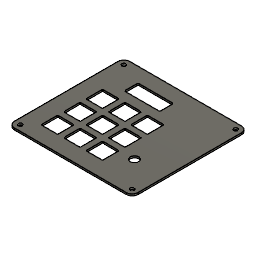
MyMacroPad (Autodesk Fusion 360 archive; units mm, degrees)
design "Top MacroPad"
Autodesk Fusion 360 part; units mm, degrees
sketch "plate-2026-01-30T15_29_04.840Z" plane through (0, 0, 0) normal (0, 0, 1) x (1, 0, 0)
  line L0 (3.025, -21.575) -> (16.025, -21.575)
  line L1 (3.025, -35.575) -> (16.025, -35.575)
  line L2 (2.525, -22.075) -> (2.525, -35.075)
  line L3 (16.525, -22.075) -> (16.525, -35.075)
  arc A0 (3.025, -21.575) -> (2.525, -22.075) centre (3.025, -22.075) ccw
  arc A1 (16.525, -22.075) -> (16.025, -21.575) centre (16.025, -22.075) ccw
  arc A2 (2.525, -35.075) -> (3.025, -35.575) centre (3.025, -35.075) ccw
  arc A3 (16.025, -35.575) -> (16.525, -35.075) centre (16.025, -35.075) ccw
  line L4 (22.075, -21.575) -> (35.075, -21.575)
  line L5 (22.075, -35.575) -> (35.075, -35.575)
  line L6 (21.575, -22.075) -> (21.575, -35.075)
  line L7 (35.575, -22.075) -> (35.575, -35.075)
  arc A4 (22.075, -21.575) -> (21.575, -22.075) centre (22.075, -22.075) ccw
  arc A5 (35.575, -22.075) -> (35.075, -21.575) centre (35.075, -22.075) ccw
  arc A6 (21.575, -35.075) -> (22.075, -35.575) centre (22.075, -35.075) ccw
  arc A7 (35.075, -35.575) -> (35.575, -35.075) centre (35.075, -35.075) ccw
  line L8 (41.125, -21.575) -> (54.125, -21.575)
  line L9 (41.125, -35.575) -> (54.125, -35.575)
  line L10 (40.625, -22.075) -> (40.625, -35.075)
  line L11 (54.625, -22.075) -> (54.625, -35.075)
  arc A8 (41.125, -21.575) -> (40.625, -22.075) centre (41.125, -22.075) ccw
  arc A9 (54.625, -22.075) -> (54.125, -21.575) centre (54.125, -22.075) ccw
  arc A10 (40.625, -35.075) -> (41.125, -35.575) centre (41.125, -35.075) ccw
  arc A11 (54.125, -35.575) -> (54.625, -35.075) centre (54.125, -35.075) ccw
  line L12 (3.025, -40.625) -> (16.025, -40.625)
  line L13 (3.025, -54.625) -> (16.025, -54.625)
  line L14 (2.525, -41.125) -> (2.525, -54.125)
  line L15 (16.525, -41.125) -> (16.525, -54.125)
  arc A12 (3.025, -40.625) -> (2.525, -41.125) centre (3.025, -41.125) ccw
  arc A13 (16.525, -41.125) -> (16.025, -40.625) centre (16.025, -41.125) ccw
  arc A14 (2.525, -54.125) -> (3.025, -54.625) centre (3.025, -54.125) ccw
  arc A15 (16.025, -54.625) -> (16.525, -54.125) centre (16.025, -54.125) ccw
  line L16 (22.075, -40.625) -> (35.075, -40.625)
  line L17 (22.075, -54.625) -> (35.075, -54.625)
  line L18 (21.575, -41.125) -> (21.575, -54.125)
  line L19 (35.575, -41.125) -> (35.575, -54.125)
  arc A16 (22.075, -40.625) -> (21.575, -41.125) centre (22.075, -41.125) ccw
  arc A17 (35.575, -41.125) -> (35.075, -40.625) centre (35.075, -41.125) ccw
  arc A18 (21.575, -54.125) -> (22.075, -54.625) centre (22.075, -54.125) ccw
  arc A19 (35.075, -54.625) -> (35.575, -54.125) centre (35.075, -54.125) ccw
  line L20 (41.125, -40.625) -> (54.125, -40.625)
  line L21 (41.125, -54.625) -> (54.125, -54.625)
  line L22 (40.625, -41.125) -> (40.625, -54.125)
  line L23 (54.625, -41.125) -> (54.625, -54.125)
  arc A20 (41.125, -40.625) -> (40.625, -41.125) centre (41.125, -41.125) ccw
  arc A21 (54.625, -41.125) -> (54.125, -40.625) centre (54.125, -41.125) ccw
  arc A22 (40.625, -54.125) -> (41.125, -54.625) centre (41.125, -54.125) ccw
  arc A23 (54.125, -54.625) -> (54.625, -54.125) centre (54.125, -54.125) ccw
  line L24 (3.025, -59.675) -> (16.025, -59.675)
  line L25 (3.025, -73.675) -> (16.025, -73.675)
  line L26 (2.525, -60.175) -> (2.525, -73.175)
  line L27 (16.525, -60.175) -> (16.525, -73.175)
  arc A24 (3.025, -59.675) -> (2.525, -60.175) centre (3.025, -60.175) ccw
  arc A25 (16.525, -60.175) -> (16.025, -59.675) centre (16.025, -60.175) ccw
  arc A26 (2.525, -73.175) -> (3.025, -73.675) centre (3.025, -73.175) ccw
  arc A27 (16.025, -73.675) -> (16.525, -73.175) centre (16.025, -73.175) ccw
  line L28 (22.075, -59.675) -> (35.075, -59.675)
  line L29 (22.075, -73.675) -> (35.075, -73.675)
  line L30 (21.575, -60.175) -> (21.575, -73.175)
  line L31 (35.575, -60.175) -> (35.575, -73.175)
  arc A28 (22.075, -59.675) -> (21.575, -60.175) centre (22.075, -60.175) ccw
  arc A29 (35.575, -60.175) -> (35.075, -59.675) centre (35.075, -60.175) ccw
  arc A30 (21.575, -73.175) -> (22.075, -73.675) centre (22.075, -73.175) ccw
  arc A31 (35.075, -73.675) -> (35.575, -73.175) centre (35.075, -73.175) ccw
  line L32 (41.125, -59.675) -> (54.125, -59.675)
  line L33 (41.125, -73.675) -> (54.125, -73.675)
  line L34 (40.625, -60.175) -> (40.625, -73.175)
  line L35 (54.625, -60.175) -> (54.625, -73.175)
  arc A32 (41.125, -59.675) -> (40.625, -60.175) centre (41.125, -60.175) ccw
  arc A33 (54.625, -60.175) -> (54.125, -59.675) centre (54.125, -60.175) ccw
  arc A34 (40.625, -73.175) -> (41.125, -73.675) centre (41.125, -73.175) ccw
  arc A35 (54.125, -73.675) -> (54.625, -73.175) centre (54.125, -73.175) ccw
  line L36 (-11.475, 10.56) -> (93.525, 10.56)
  line L37 (93.525, 10.56) -> (93.525, -87.44)
  line L38 (93.525, -87.44) -> (-11.475, -87.44)
  line L39 (-11.475, -87.44) -> (-11.475, 10.56)
  line L40 (13.025, -1.94) -> (43.025, -1.94)
  line L41 (43.025, -1.94) -> (43.025, -13.44)
  line L42 (43.025, -13.44) -> (13.025, -13.44)
  line L43 (13.025, -13.44) -> (13.025, -1.94)
  circle A36 centre (67.525, -59.44) radius 3.55
  circle A37 centre (-6.475, -82.44) radius 1.7
  circle A38 centre (-6.475, 5.56) radius 1.7
  circle A39 centre (88.525, 5.56) radius 1.7
  circle A40 centre (88.525, -82.44) radius 1.7
  dimension "d1" = 98
  dimension "d2" = 105
  dimension "d4" = 14
  dimension "d5" = 13.765
  dimension "d9" = 12.5
  dimension "d13" = 7.1
  dimension "d16" = 3.4
  dimension "d17" = 5
  dimension "d18" = 5
  dimension "d19" = 3.4
  dimension "d20" = 5
  dimension "d21" = 5
  dimension "d22" = 3.4
  dimension "d23" = 5
  dimension "d24" = 5
  dimension "d25" = 3.4
  dimension "d26" = 5
  dimension "d27" = 5
  dimension "d28" = 30
  dimension "d29" = 11.5
  dimension "d56" = 24.5
  dimension "d63" = 28
  dimension "d64" = 26
  constraint horizontal L36
  constraint vertical L37
  constraint horizontal L38
  constraint vertical L39
  constraint horizontal L40
  constraint vertical L41
  constraint horizontal L42
  constraint vertical L43
  measures "d1" distance of L36.start L38.end
  measures "d2" distance of L36.start L36.end
  measures "d4" distance of L26.start L39
  measures "d5" distance of L25.start L38
  measures "d9" distance of L36 L40.start
  measures "d13" diameter of A36
  measures "d16" diameter of A37
  measures "d17" distance of L38 A37.centre
  measures "d18" distance of L39 A37.centre
  measures "d19" diameter of A38
  measures "d20" distance of L36 A38.centre
  measures "d21" distance of L39 A38.centre
  measures "d22" diameter of A39
  measures "d23" distance of L36 A39.centre
  measures "d24" distance of L37 A39.centre
  measures "d25" diameter of A40
  measures "d26" distance of L38 A40.centre
  measures "d27" distance of L37 A40.centre
  measures "d28" distance of L40.start L40.end
  measures "d29" distance of L40.start L42.end
  measures "d56" distance of L39 L42.end
  measures "d63" distance of L38 A36.centre
  measures "d64" distance of L37 A36.centre
extrude "Extrude1" add sketch "plate-2026-01-30T15_29_04.840Z" along normal blind 3
fillet "Fillet1" radius 5 1 edges at (93.525, 10.56, 1.5)
fillet "Fillet2" radius 5 1 edges at (93.525, -87.44, 1.5)
fillet "Fillet3" radius 5 1 edges at (-11.475, -87.44, 1.5)
fillet "Fillet4" radius 5 1 edges at (-11.475, 10.56, 1.5)
fillet "Fillet5" radius 1 1 edges at (43.025, -13.44, 1.5)
fillet "Fillet6" radius 1 1 edges at (13.025, -1.94, 1.5)
fillet "Fillet7" radius 1 1 edges at (43.025, -1.94, 1.5)
fillet "Fillet8" radius 1 1 edges at (13.025, -13.44, 1.5)
extrude "Extrude2" cut 1 faces at (85.9245, -44.9266, 3) along direction (0, 0, -1) blind 1.5
sketch "Sketch2" plane through (0, 0, 0) normal (0, 0, -1) x (1, 0, 0)
  circle A0 centre (67.525, 59.44) radius 3.55
  arc A1 (21.575, 41.125) -> (22.075, 40.625) centre (22.075, 41.125) ccw
  line L0 (21.575, 41.125) -> (21.575, 54.125)
  arc A2 (22.075, 54.625) -> (21.575, 54.125) centre (22.075, 54.125) ccw
  line L1 (22.075, 54.625) -> (35.075, 54.625)
  arc A3 (35.575, 54.125) -> (35.075, 54.625) centre (35.075, 54.125) ccw
  line L2 (35.575, 54.125) -> (35.575, 41.125)
  arc A4 (35.075, 40.625) -> (35.575, 41.125) centre (35.075, 41.125) ccw
  line L3 (35.075, 40.625) -> (22.075, 40.625)
  circle A5 centre (88.525, -5.56) radius 1.7
  arc A6 (2.525, 60.175) -> (3.025, 59.675) centre (3.025, 60.175) ccw
  line L4 (2.525, 60.175) -> (2.525, 73.175)
  arc A7 (3.025, 73.675) -> (2.525, 73.175) centre (3.025, 73.175) ccw
  line L5 (3.025, 73.675) -> (16.025, 73.675)
  arc A8 (16.525, 73.175) -> (16.025, 73.675) centre (16.025, 73.175) ccw
  line L6 (16.525, 73.175) -> (16.525, 60.175)
  arc A9 (16.025, 59.675) -> (16.525, 60.175) centre (16.025, 60.175) ccw
  line L7 (16.025, 59.675) -> (3.025, 59.675)
  arc A10 (40.625, 22.075) -> (41.125, 21.575) centre (41.125, 22.075) ccw
  line L8 (40.625, 22.075) -> (40.625, 35.075)
  arc A11 (41.125, 35.575) -> (40.625, 35.075) centre (41.125, 35.075) ccw
  line L9 (41.125, 35.575) -> (54.125, 35.575)
  arc A12 (54.625, 35.075) -> (54.125, 35.575) centre (54.125, 35.075) ccw
  line L10 (54.625, 35.075) -> (54.625, 22.075)
  arc A13 (54.125, 21.575) -> (54.625, 22.075) centre (54.125, 22.075) ccw
  line L11 (54.125, 21.575) -> (41.125, 21.575)
  arc A14 (21.575, 22.075) -> (22.075, 21.575) centre (22.075, 22.075) ccw
  line L12 (21.575, 22.075) -> (21.575, 35.075)
  arc A15 (22.075, 35.575) -> (21.575, 35.075) centre (22.075, 35.075) ccw
  line L13 (22.075, 35.575) -> (35.075, 35.575)
  arc A16 (35.575, 35.075) -> (35.075, 35.575) centre (35.075, 35.075) ccw
  line L14 (35.575, 35.075) -> (35.575, 22.075)
  arc A17 (35.075, 21.575) -> (35.575, 22.075) centre (35.075, 22.075) ccw
  line L15 (35.075, 21.575) -> (22.075, 21.575)
  arc A18 (21.575, 60.175) -> (22.075, 59.675) centre (22.075, 60.175) ccw
  line L16 (21.575, 60.175) -> (21.575, 73.175)
  arc A19 (22.075, 73.675) -> (21.575, 73.175) centre (22.075, 73.175) ccw
  line L17 (22.075, 73.675) -> (35.075, 73.675)
  arc A20 (35.575, 73.175) -> (35.075, 73.675) centre (35.075, 73.175) ccw
  line L18 (35.575, 73.175) -> (35.575, 60.175)
  arc A21 (35.075, 59.675) -> (35.575, 60.175) centre (35.075, 60.175) ccw
  line L19 (35.075, 59.675) -> (22.075, 59.675)
  circle A22 centre (-6.475, 82.44) radius 1.7
  arc A23 (40.625, 60.175) -> (41.125, 59.675) centre (41.125, 60.175) ccw
  line L20 (40.625, 60.175) -> (40.625, 73.175)
  arc A24 (41.125, 73.675) -> (40.625, 73.175) centre (41.125, 73.175) ccw
  line L21 (41.125, 73.675) -> (54.125, 73.675)
  arc A25 (54.625, 73.175) -> (54.125, 73.675) centre (54.125, 73.175) ccw
  line L22 (54.625, 73.175) -> (54.625, 60.175)
  arc A26 (54.125, 59.675) -> (54.625, 60.175) centre (54.125, 60.175) ccw
  line L23 (54.125, 59.675) -> (41.125, 59.675)
  circle A27 centre (-6.475, -5.56) radius 1.7
  circle A28 centre (88.525, 82.44) radius 1.7
  arc A29 (40.625, 41.125) -> (41.125, 40.625) centre (41.125, 41.125) ccw
  line L24 (40.625, 41.125) -> (40.625, 54.125)
  arc A30 (41.125, 54.625) -> (40.625, 54.125) centre (41.125, 54.125) ccw
  line L25 (41.125, 54.625) -> (54.125, 54.625)
  arc A31 (54.625, 54.125) -> (54.125, 54.625) centre (54.125, 54.125) ccw
  line L26 (54.625, 54.125) -> (54.625, 41.125)
  arc A32 (54.125, 40.625) -> (54.625, 41.125) centre (54.125, 41.125) ccw
  line L27 (54.125, 40.625) -> (41.125, 40.625)
  arc A33 (2.525, 41.125) -> (3.025, 40.625) centre (3.025, 41.125) ccw
  line L28 (2.525, 41.125) -> (2.525, 54.125)
  arc A34 (3.025, 54.625) -> (2.525, 54.125) centre (3.025, 54.125) ccw
  line L29 (3.025, 54.625) -> (16.025, 54.625)
  arc A35 (16.525, 54.125) -> (16.025, 54.625) centre (16.025, 54.125) ccw
  line L30 (16.525, 54.125) -> (16.525, 41.125)
  arc A36 (16.025, 40.625) -> (16.525, 41.125) centre (16.025, 41.125) ccw
  line L31 (16.025, 40.625) -> (3.025, 40.625)
  arc A37 (43.025, 12.44) -> (42.025, 13.44) centre (42.025, 12.44) ccw
  line L32 (43.025, 12.44) -> (43.025, 2.94)
  arc A38 (42.025, 1.94) -> (43.025, 2.94) centre (42.025, 2.94) ccw
  line L33 (42.025, 1.94) -> (14.025, 1.94)
  arc A39 (13.025, 2.94) -> (14.025, 1.94) centre (14.025, 2.94) ccw
  line L34 (13.025, 2.94) -> (13.025, 12.44)
  arc A40 (14.025, 13.44) -> (13.025, 12.44) centre (14.025, 12.44) ccw
  line L35 (14.025, 13.44) -> (42.025, 13.44)
  arc A41 (2.525, 22.075) -> (3.025, 21.575) centre (3.025, 22.075) ccw
  line L36 (2.525, 22.075) -> (2.525, 35.075)
  arc A42 (3.025, 35.575) -> (2.525, 35.075) centre (3.025, 35.075) ccw
  line L37 (3.025, 35.575) -> (16.025, 35.575)
  arc A43 (16.525, 35.075) -> (16.025, 35.575) centre (16.025, 35.075) ccw
  line L38 (16.525, 35.075) -> (16.525, 22.075)
  arc A44 (16.025, 21.575) -> (16.525, 22.075) centre (16.025, 22.075) ccw
  line L39 (16.025, 21.575) -> (3.025, 21.575)
  arc A45 (-11.475, -5.56) -> (-6.475, -10.56) centre (-6.475, -5.56) ccw
  line L40 (-6.475, -10.56) -> (88.525, -10.56)
  arc A46 (88.525, -10.56) -> (93.525, -5.56) centre (88.525, -5.56) ccw
  line L41 (93.525, -5.56) -> (93.525, 82.44)
  arc A47 (93.525, 82.44) -> (88.525, 87.44) centre (88.525, 82.44) ccw
  line L42 (88.525, 87.44) -> (-6.475, 87.44)
  arc A48 (-6.475, 87.44) -> (-11.475, 82.44) centre (-6.475, 82.44) ccw
  line L43 (-11.475, 82.44) -> (-11.475, -5.56)
  line L44 (75.3414, 10.4867) -> (60.3414, 10.4867) construction
  line L45 (60.3414, 10.4867) -> (60.3414, 1.4867) construction
  line L46 (60.3414, 1.4867) -> (75.3414, 1.4867) construction
  line L47 (75.3414, 1.4867) -> (75.3414, 10.4867) construction
  dimension "d50" = 3
  text T0 "My MacroPad" font "Arial" height 3 align left top in box 15 x 9 at (75.3414, 10.4867) x (-1, 0) y (0, -1) spacing 1 kerned
extrude "Extrude3" cut sketch "Sketch2" against normal blind 0.2 text T0
equation "d51 = 'My MacroPad'"
